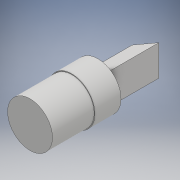
# Autodesk Inventor part: TriangleAdapter
Saved by Autodesk Inventor 2017 (Build 210142000, 142)
## iProperties
Created: 2017-03-02
Part Number: TriangleAdapter
Material: Generic
Document SubType Name: Modeling
Designer: aribu
Density: 1 g/cm^3
Appearance: Default
Author: aribu
Autodesk Inventor part; units mm, degrees
ref_plane "YZ Plane" through (0, 0, 0) normal (1, 0, 0) x (0, 1, 0)
ref_plane "XZ Plane" through (0, 0, 0) normal (0, 1, 0) x (-1, 0, 0)
ref_plane "XY Plane" through (0, 0, 0) normal (0, 0, 1) x (1, 0, 0)
sketch "Sketch1" plane through (0, 0, 0) normal (0, 1, 0) x (-1, 0, 0)
  circle A0 centre (0, 0) radius 4.3
  dimension "d0" = 8.6
  constraints: 1 centre point, 1 coincident
  measures "d0" diameter of A0
extrude "Extrusion1" add sketch "Sketch1" along normal blind 8
sketch "Sketch2" plane through (0, 8, 0) normal (0, 1, 0) x (1, 0, 0)
  circle A0 centre (0, 0) radius 4.45
  dimension "d3" = 8.9
  constraints: 1 centre point, 1 coincident
  measures "d3" diameter of A0
extrude "Extrusion2" add sketch "Sketch2" along normal blind 5
sketch "Sketch3" plane through (0, 13, 0) normal (0, 1, 0) x (1, 0, 0)
  line L0 (-3.4193, -0.0029) -> (1.6902, -2.9529)
  line L1 (1.6902, -2.9529) -> (1.6902, 2.9471)
  line L2 (1.6902, 2.9471) -> (-3.4193, -0.0029)
  point P0 (0, 0)
  dimension "d6" = 5.9
  dimension "d7" = 5.9
  dimension "d8" = 5.9
  constraints: 6 end point, 1 vertical
  measures "d6" distance of L0.start L0.end
  measures "d7" distance of L1.end L0.start
  measures "d8" distance of L0.end L1.end
extrude "Extrusion3" add sketch "Sketch3" along normal blind 10
equation "\"d7\" = d6"
equation "\"d8\" = d6"
body "Solid1"
